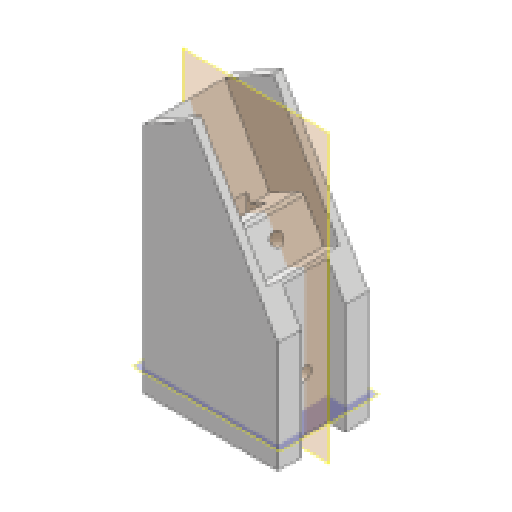
# Autodesk Inventor part: PALM 4
Saved by Autodesk Inventor 2025 (Build 290162010, 162A)
## iProperties
Created: 2024-12-04
Part Number: PALM 4
Material: Generic
Document SubType Name: Modeling
Designer: ALEXANDERNICHOLS
Density: 1 g/cm^3
Appearance: Default
Mass: 40.9753 g
Surface Area: 126.071 cm^2
Volume: 40.9753 cm^3
Author: ALEXANDERNICHOLS
Autodesk Inventor part; units mm, degrees
ref_plane "YZ Plane" through (0, 0, 0) normal (1, 0, 0) x (0, 1, 0)
ref_plane "XZ Plane" through (0, 0, 0) normal (0, 1, 0) x (-1, 0, 0)
sketch "Sketch1" plane through (0, 0, 0) normal (0, 0, 1) x (1, 0, 0)
  line L0 (0, 0) -> (38.1, 0)
  line L1 (38.1, 0) -> (38.1, 31.4433)
  line L2 (0, 66.04) -> (0, 0)
  line L3 (0, 66.04) -> (13.5942, 73.8886)
  line L4 (0, 66.04) -> (12.7, 44.043)
  line L5 (12.7, 44.043) -> (26.2942, 51.8916)
  line L6 (26.2942, 51.8916) -> (13.5942, 73.8886)
  line L7 (26.2942, 51.8916) -> (38.1, 31.4433)
  dimension "d0" = 15.6972
  dimension "d1" = 25.4
  dimension "d2" = 38.1
  dimension "d3" = 66.04
  dimension "d4" = 120
  constraints: 16 end point, 4 perpendicular, 2 point on line, 1 collinear, 1 horizontal, 1 parallel
  measures "d0" distance between parallel lines of L4 L6
  measures "d1" distance between parallel lines of L5 L3
  measures "d2" distance of L0.start L0.end
  measures "d3" distance from line of L2.start L0
  measures "d4" angle of L2 L3
extrude "Extrusion1" add sketch "Sketch1" along normal blind 20.574 contours L2 L4 L5 L7 L1 L0
sketch "Sketch2" plane through (0, 0, 20.574) normal (0, 0, 1) x (1, 0, 0)
  line L0 (0, 66.04) -> (0, 0) projected
  line L1 (0, 0) -> (38.1, 0) projected
  line L2 (38.1, 0) -> (38.1, 31.4433) projected
  line L3 (38.1, 31.4433) -> (26.2942, 51.8916) projected
  line L4 (26.2942, 51.8916) -> (12.7, 44.043) projected
  line L5 (12.7, 44.043) -> (0, 66.04) projected
  line L6 (26.2942, 51.8916) -> (13.5942, 73.8886)
  line L7 (13.5942, 73.8886) -> (0, 66.04)
  line L8 (38.1, 31.4433) -> (26.2942, 51.8916) projected
  constraints: 4 end point, 1 collinear, 1 perpendicular
extrude "Extrusion2" add sketch "Sketch2" along normal blind 2.54
ref_plane "Work Plane1" through (0, 0, 10.287) normal (0, 0, -1) x (-1, 0, 0)
mirror "Mirror1" about plane through (0, 0, 10.287) normal (0, 0, -1) of "Extrusion2"
sketch "Sketch3" plane through (0, 0, 23.114) normal (0, -1, 0) x (1, 0, 0)
  line L0 (38.1, -25.654) -> (38.1, 0) projected
  line L1 (38.1, -6.477) -> (33.02, -6.477)
  line L2 (33.02, -6.477) -> (33.02, -19.177)
  line L3 (33.02, -19.177) -> (38.1, -19.177)
  line L4 (38.1, -19.177) -> (38.1, -6.477)
  point P0 (0, -23.114)
  point P1 (38.1, -12.827)
  dimension "d9" = 12.7
  dimension "d10" = 5.08
  dimension "d11" = 6.35
  constraints: 8 end point, 2 parallel, 1 horizontal, 1 midpoint, 1 perpendicular, 1 point on line
  measures "d9" distance between parallel lines of L3 L1
  measures "d10" distance between parallel lines of L0 L2
  measures "d11" distance from line of point (38.1, -12.827) L3
extrude "Extrusion3" cut sketch "Sketch3" against normal blind 111.125
sketch "Sketch4" plane through (33.02, 0, 16.637) normal (1, 0, 0) x (0, 0, -1)
  circle A0 centre (6.35, 15.042) radius 1.778 projected
  point P0 (16.637, 0)
extrude "Extrusion4" cut sketch "Sketch4" against normal blind 15.24
sketch "Sketch5" plane through (13.5942, 73.8886, 23.114) normal (0.8660254, 0.5, 0) x (0, 0, -1)
  line L0 (23.114, -25.4) -> (2.54, -25.4) projected
  line L1 (23.114, -25.4) -> (2.54, -25.4)
  line L2 (2.54, -25.4) -> (2.54, -37.7698)
  line L3 (2.54, -37.7698) -> (23.114, -37.7698)
  line L4 (23.114, -37.7698) -> (23.114, -25.4)
  point P0 (23.114, -57.1923)
  dimension "d16" = 12.3698
  constraints: 8 end point, 2 parallel, 1 horizontal, 1 perpendicular
  measures "d16" distance between parallel lines of L0 L3
extrude "Extrusion5" cut sketch "Sketch5" against normal blind 5.08
chamfer "Chamfer1" distance 1.016 angle 45 1 edges at (21.893, 49.3506, 10.287)
sketch "Sketch6" plane through (9.1948, 71.3486, 23.114) normal (0.8660254, 0.5, 0) x (0, 0, -1)
  line L0 (22.86, -25.4) -> (2.54, -25.4) projected
  line L1 (23.114, -37.7698) -> (2.54, -37.7698) projected
  line L2 (2.54, -25.4) -> (2.54, 0) projected
  line L3 (2.54, -37.7698) -> (2.54, 0) projected
  line L4 (2.54, -25.4) -> (2.54, -37.7698)
  circle A0 centre (12.827, -31.5849) radius 1.778
  point P0 (23.114, -57.1923)
  point P1 (2.54, -31.5849)
  point P2 (12.827, -37.7698)
  dimension "d22" = 3.556
  constraints: 2 end point, 2 midpoint, 1 centre point, 1 collinear, 1 horizontal alignment, 1 vertical alignment
  measures "d22" diameter of A0
extrude "Extrusion6" cut sketch "Sketch6" against normal blind 7.62
ref_plane "Work Plane2" through (0, 0, 10.287) normal (0, 0, 1) x (1, 0, 0)
sketch "Sketch7" plane through (0, 0, 10.287) normal (0, 0, 1) x (1, 0, 0)
  line L0 (12.7, 44.043) -> (-2.54, 70.4394) projected
  line L1 (21.0809, 48.8817) -> (12.7, 44.043) projected
  line L2 (16.51, 46.2427) -> (11.43, 46.2427)
  line L3 (11.43, 46.2427) -> (11.43, 0)
  line L4 (11.43, 0) -> (16.51, 0)
  line L5 (16.51, 0) -> (16.51, 46.2427)
  line L6 (0, 0) -> (38.1, 0) projected
  dimension "d25" = 5.08
  constraints: 8 end point, 3 point on line, 2 parallel, 1 horizontal, 1 perpendicular
  measures "d25" distance between parallel lines of L5 L3
extrude "Extrusion7" cut sketch "Sketch7" along normal mid plane 10.16 contours L1 L5 L4 L3 L0
ref_plane "Work Plane3" through (0, 6.35, 23.114) normal (0, -1, 0) x (1, 0, 0)
sketch "Sketch8" plane through (0, 6.35, 23.114) normal (0, -1, 0) x (1, 0, 0)
  line L0 (0, -25.654) -> (38.1, -25.654) projected
  line L1 (0, -25.654) -> (0, 0) projected
  line L2 (14.7303, -25.654) -> (17.0826, -23.0077)
  line L3 (17.0826, -23.0077) -> (0, -7.8232)
  line L4 (4.8537, -36.7652) -> (14.7303, -25.654) projected
  line L5 (0, -32.4508) -> (-19.3376, -15.2619) projected
  point P0 (0, -23.114)
  dimension "d37" = 17.8308
  constraints: 4 end point, 2 point on line, 1 collinear, 1 parallel
  measures "d37" distance from line of L3.end L0
extrude "Extrusion8" cut sketch "Sketch8" against normal blind 12.7
sketch "Sketch9" plane through (0, 6.35, 15.2908) normal (-0.6643638, 0, -0.7474093) x (-0.7474093, 0, 0.6643638)
  line L0 (-8.4923, 39.8927) -> (-8.4923, -6.35) projected
  line L1 (-19.039, 39.8927) -> (-19.039, -6.35) projected
  line L2 (-22.8557, 0) -> (0, 0) projected
  line L3 (0, 12.7) -> (-22.8557, 12.7) projected
  point P0 (-10.1587, -6.35)
  point P1 (-8.4923, 12.7)
  point P2 (-19.039, 12.7)
  point P3 (-19.039, 0)
  point P4 (-8.4923, 0)
extrude "Extrusion9" cut sketch "Sketch9" against normal up to next
sketch "Sketch11" plane through (0, 0, 23.114) normal (-1, 0, 0) x (0, 0, 1)
  circle A0 centre (-12.827, 35.56) radius 1.778 projected
  point P0 (-23.114, 0)
extrude "Extrusion11" cut sketch "Sketch11" against normal blind 15.24
sketch "Sketch13" plane through (0, 0, 23.114) normal (0, -1, 0) x (1, 0, 0)
  circle A0 centre (22.86, -6.35) radius 1.778 projected
  point P0 (0, -23.114)
extrude "Extrusion13" cut sketch "Sketch13" against normal blind 15.24
sketch "Sketch14" plane through (38.1, 0, -2.54) normal (0, 0, -1) x (-1, 0, 0)
  circle A0 centre (12.7, 25.4) radius 1.778 projected
  point P0 (38.1, 0)
extrude "Extrusion14" cut sketch "Sketch14" against normal blind 15.24
sketch "Sketch15" plane through (0, 0, 5.207) normal (0, 0, 1) x (1, 0, 0)
  line L0 (16.51, 6.35) -> (16.51, 0) projected
  line L1 (11.43, 0) -> (16.51, 0)
  line L2 (16.51, 0) -> (16.51, 7.62)
  line L3 (16.51, 7.62) -> (11.43, 7.62)
  line L4 (11.43, 7.62) -> (11.43, 0)
  point P0 (0, 0)
  dimension "d50" = 7.62
  constraints: 8 end point, 2 parallel, 1 horizontal, 1 perpendicular, 1 point on line
  measures "d50" distance between parallel lines of L1 L3
extrude "Extrusion15" cut sketch "Sketch15" against normal blind 12.7
equation "\"d11\" = 0.5 * d9"
body "Solid1"
